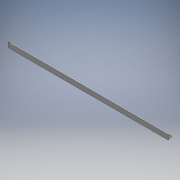
# Autodesk Inventor part: junta controler2
Saved by Autodesk Inventor 2016 (Build 200138000, 138)
## iProperties
Created: 2017-06-07
Part Number: junta controler2
Material: Generic
Document SubType Name: Modeling
Designer: fabio-note
Density: 1 g/cm^3
Appearance: Default
Author: fabio-note
Autodesk Inventor part; units mm, degrees
ref_plane "YZ Plane" through (0, 0, 0) normal (1, 0, 0) x (0, 1, 0)
ref_plane "XZ Plane" through (0, 0, 0) normal (0, 1, 0) x (-1, 0, 0)
ref_plane "XY Plane" through (0, 0, 0) normal (0, 0, 1) x (1, 0, 0)
sketch "Sketch1" plane through (0, 0, 0) normal (1, 0, 0) x (0, 1, 0)
  line L0 (5, -15.415) -> (5, -19.415)
  line L1 (5, -20.415) -> (8.7898, -19.1353)
  arc A0 (8.7898, -19.1353) -> (5, -15.415) centre (1.7532, -22.5129) ccw
  line L2 (5, -19.415) -> (5, -20.415)
  point P0 (0, 0)
  point P1 (0, -20.415)
  dimension "d0" = 4
  dimension "d4" = 4
  constraints: 6 end point, 2 point on circle, 2 vertical, 1 centre point, 1 vertical alignment
  measures "d0" distance of L0.start L0.end
  measures "d4" distance of L1.end L1.start
extrude "Extrusion1" add sketch "Sketch1" along normal blind 165
body "Solid1"
